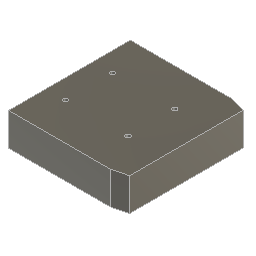
Крепление аккамулятора GreenWorks (Autodesk Fusion 360 design; units mm, degrees)
Autodesk Fusion 360 part; units mm, degrees
sketch "Sketch1" plane through (0, 0, 0) normal (0, 0, 1) x (1, 0, 0)
  line L0 (27.5, 28) -> (-37.5, 28)
  line L1 (-37.5, 39) -> (-37.5, -23.5)
  line L2 (-37.5, -28) -> (27.5, -28)
  line L3 (27.5, -28) -> (27.5, 28)
  line L4 (27.5, 23.5) -> (-37.5, 23.5)
  line L5 (-37.5, -23.5) -> (27.5, -23.5)
  line L6 (27.5, -23.5) -> (27.5, 23.5)
  line L7 (27.5, 39) -> (-37.5, 39)
  line L8 (37.5, -28) -> (37.5, 36.48)
  line L9 (27.5, 39) -> (37.5, 36.48)
  line L10 (1.75, 0) -> (22.5, 0)
  line L11 (37.5, 28) -> (37.5, -36.48)
  line L12 (27.5, -39) -> (37.5, -36.48)
  line L13 (27.5, -39) -> (-37.5, -39)
  line L14 (-37.5, -39) -> (-37.5, 23.5)
  dimension "d1" = 65
  dimension "d2" = 56
  dimension "d3" = 65
  dimension "d4" = 47
  dimension "d5" = 11
  dimension "d6" = 10
  constraint horizontal L0
  constraint perpendicular L0 L1
  constraint parallel L0 L2
  constraint parallel L1 L3
  constraint horizontal L4
  constraint perpendicular L1 L4
  constraint parallel L4 L5
  constraint parallel L1 L6
  constraint coincident L0.end L1
  constraint symmetric L1.end L10 L4.end
  constraint symmetric L7.start L10 L12.start
  constraint symmetric L1.start L10 L13.end
  constraint symmetric L8.start L10 L11.start
  constraint symmetric L8.end L10 L11.end
  measures "d1" distance of L2.start L2.end
  measures "d2" distance of L0.end L2.start
  measures "d3" distance of L1.end L5.end
  measures "d4" distance of L4.end L1.end
extrude "Extrude1" add sketch "Sketch1" along normal blind 5.8 contours L0 L1 L3 L4 | L0 L1 L2 L3 L6 L7 L8 L9 L11 L12 L13 L14 | L2 L3 L5 L14
extrude "Extrude2" add sketch "Sketch1" along normal blind 17 contours L0 L1 L2 L3 L6 L7 L8 L9 L11 L12 L13 L14
extrude "Extrude3" add sketch "Sketch1" along normal blind 21 and the other way blind -17
sketch "Sketch2" plane through (0, 0, 21) normal (0, 0, 1) x (-1, 0, 0)
  line L0 (37.5, -39) -> (37.5, 39)
  line L1 (37.5, 39) -> (-27.5, 39)
  line L2 (-27.5, 39) -> (-37.5, 36.48)
  line L3 (-37.5, 36.48) -> (-37.5, -36.48)
  line L4 (-37.5, -36.48) -> (-27.5, -39)
  line L5 (-27.5, -39) -> (37.5, -39)
  circle A0 centre (25, 15) radius 1.5
  circle A1 centre (-15, 15) radius 1.5
  line L6 (-1.75, 0) -> (-22.5, 0)
  circle A2 centre (25, -15) radius 1.5
  circle A3 centre (-15, -15) radius 1.5
  dimension "d15" = 3
  dimension "d16" = 3
  constraint symmetric A0 L6 A2
  constraint symmetric A1 L6 A3
  measures "d15" diameter of A0
  measures "d16" diameter of A1
extrude "Extrude4" cut sketch "Sketch2" against normal blind 5 contours A0 | A1 | A2 | A3
chamfer "Chamfer1" distance 1 angle 45 4 edges at (-23.6015, 15.5424, 17) (-23.6015, -14.4576, 17) (16.3985, -14.4576, 17) (16.3985, 15.5424, 17)
